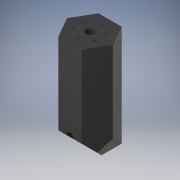
# Autodesk Inventor part: TARM01
Saved by Autodesk Inventor 2017 (Build 210142000, 142)
## iProperties
Created: 2018-10-11
Part Number: TARM01
Material: ABS Plastic
Document SubType Name: Modeling
Designer: Zach
Density: 1.06 g/cm^3
Appearance: Smooth - Black
Author: Zach
Autodesk Inventor part; units mm, degrees
ref_plane "YZ Plane" through (0, 0, 0) normal (1, 0, 0) x (0, 1, 0)
ref_plane "XZ Plane" through (0, 0, 0) normal (0, 1, 0) x (-1, 0, 0)
ref_plane "XY Plane" through (0, 0, 0) normal (0, 0, 1) x (1, 0, 0)
sketch "Sketch9" plane through (0, 0, 0) normal (0, 0, 1) x (1, 0, 0)
  line L0 (56, 0) -> (28, -48.4974)
  line L1 (28, -48.4974) -> (-28, -48.4974)
  line L2 (-28, -48.4974) -> (-56, 0)
  line L3 (-56, 0) -> (-28, 48.4974)
  line L4 (-28, 48.4974) -> (28, 48.4974)
  line L5 (28, 48.4974) -> (56, 0)
  circle A0 centre (25.9808, 15) radius 2.5
  circle A1 centre (0, 0) radius 10
  circle A2 centre (0, 30) radius 2.5
  circle A3 centre (-25.9808, 15) radius 2.5
  circle A4 centre (-25.9808, -15) radius 2.5
  circle A5 centre (0, -30) radius 2.5
  circle A6 centre (25.9808, -15) radius 2.5
  dimension "d52" = 112
  dimension "d53" = 5
  dimension "d54" = 30
  dimension "d55" = 20
  dimension "d58" = 360
  constraints: 12 end point, 7 centre point, 2 coincident, 1 horizontal alignment, 1 vertical alignment, 26 other
  measures "d52" distance of L0.start L2.end
  measures "d53" diameter of A0
  measures "d54" distance of A0.centre point (0, 0)
  measures "d55" diameter of A1
extrude "Extrusion7" add sketch "Sketch9" along normal blind 96.995
sketch "Sketch10" plane through (0, 0, 96.995) normal (0, 0, 1) x (1, 0, 0)
  line L0 (28, -48.4974) -> (56, 0) projected
  line L1 (56, 0) -> (56, 48.4974)
  line L2 (28, 48.4974) -> (-28, 48.4974) projected
  line L3 (56, 48.4974) -> (28, 48.4974)
  line L4 (-28, 48.4974) -> (-56, 0) projected
  line L5 (-56, 0) -> (-56, 48.4974)
  line L6 (-56, 48.4974) -> (-28, 48.4974)
  line L7 (56, 0) -> (28, 48.4974) projected
  point P0 (0, 0)
  constraints: 8 end point, 2 perpendicular, 2 vertical
extrude "Extrusion8" add sketch "Sketch10" against normal blind 96.995
sketch "Sketch11" plane through (-56, 48.4974, 0) normal (0, 1, 0) x (1, 0, 0)
  line L0 (112.0001, -48.4975) -> (84, -96.995)
  line L1 (84, -96.995) -> (28, -96.995)
  line L2 (28, -96.995) -> (-0.0001, -48.4975)
  line L3 (-0.0001, -48.4975) -> (28, 0)
  line L4 (28, 0) -> (84, 0)
  line L5 (84, 0) -> (112.0001, -48.4975)
  line L6 (0, 0) -> (112, 0) projected
  line L7 (0, -96.995) -> (0, 0) projected
  line L8 (112, -96.995) -> (0, -96.995) projected
  line L9 (112, -96.995) -> (112, 0) projected
  line L10 (0, -96.995) -> (0, 0) projected
  line L11 (-0.0001, -48.4975) -> (0, -96.995)
  line L12 (0, -96.995) -> (0, -96.995)
  line L13 (112, -96.995) -> (0, -96.995) projected
  line L14 (28, -96.995) -> (0, -96.995)
  line L15 (0, 0) -> (112, 0) projected
  line L16 (-0.0001, -48.4975) -> (0, 0)
  line L17 (0, 0) -> (28, 0)
  line L18 (84, 0) -> (112, 0)
  line L19 (112, 0) -> (112.0001, -48.4975)
  line L20 (112.0001, -48.4975) -> (112, -96.995)
  line L21 (112, -96.995) -> (84, -96.995)
  point P0 (56, -48.4975)
  point P1 (56, 0)
  constraints: 30 end point, 3 horizontal alignment, 2 collinear, 2 midpoint, 1 horizontal, 13 other
extrude "Extrusion9" cut sketch "Sketch11" against normal through all contours L9 L8 L0 | L5 L6 L9 | L8 L7 L2 | L3 L7 L6
sketch "Sketch12" plane through (-28, 48.4974, 96.995) normal (0, 1, 0) x (1, 0, 0)
  circle A0 centre (28, 48.4973) radius 10
  line L0 (0, 96.995) -> (56.0001, 96.995) projected
  circle A1 centre (28, 78.4973) radius 2.5
  circle A2 centre (2.0193, 63.4973) radius 2.5
  circle A3 centre (2.0193, 33.4973) radius 2.5
  circle A4 centre (28, 18.4973) radius 2.5
  circle A5 centre (53.9808, 33.4973) radius 2.5
  circle A6 centre (53.9808, 63.4973) radius 2.5
  point P0 (28, 96.995)
  point P1 (28, 96.995)
  point P2 (84, 48.4973)
  dimension "d66" = 20
  dimension "d67" = 5
  dimension "d68" = 30
  dimension "d71" = 360
  constraints: 7 centre point, 2 vertical alignment, 1 horizontal alignment, 1 midpoint, 13 other
  measures "d66" diameter of A0
  measures "d67" diameter of A1
  measures "d68" distance of A0.centre A1.centre
extrude "Extrusion10" cut sketch "Sketch12" against normal through all
chamfer "Chamfer2" distance 48.4973 angle 45 1 edges at (0, -48.4974, 96.995)
sketch "Sketch14" plane through (-28, 48.4974, 96.995) normal (0, 1, 0) x (1, 0, 0)
  circle A0 centre (53.9808, 63.4973) radius 2.5 projected
  circle A1 centre (28, 18.4973) radius 2.5 projected
  circle A2 centre (2.0193, 63.4973) radius 2.5 projected
  circle A3 centre (28, 78.4973) radius 2.5 projected
  circle A4 centre (2.0193, 33.4973) radius 2.5 projected
  circle A5 centre (53.9808, 33.4973) radius 2.5 projected
  circle A6 centre (28, 48.4973) radius 10 projected
  line L0 (0, 96.995) -> (-28, 48.4977) projected
  line L1 (-28, 48.4973) -> (-28, 48.4977) projected
  line L2 (-28, 48.4973) -> (0, 0) projected
  line L3 (56.0001, 0) -> (0, 0) projected
  line L4 (56.0001, 0) -> (84, 48.4973) projected
  line L5 (84, 48.4973) -> (84, 48.4977) projected
  line L6 (84, 48.4977) -> (56.0001, 96.995) projected
  line L7 (0, 96.995) -> (56.0001, 96.995) projected
  point P0 (28, 96.995)
extrude "Extrusion12" add sketch "Sketch14" along normal blind 150
body "Solid2"
